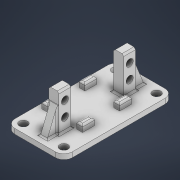
# Autodesk Inventor part: Servo mount
Saved by Autodesk Inventor 2021 (Build 250183000, 183)
## iProperties
Created: 2021-04-20
Part Number: Servo mount
Material: Generic
Document SubType Name: Modeling
Designer: allen
Density: 1 g/cm^3
Appearance: Default
Author: allen
Autodesk Inventor part; units mm, degrees
ref_plane "YZ Plane" through (0, 0, 0) normal (1, 0, 0) x (0, 1, 0)
ref_plane "XZ Plane" through (0, 0, 0) normal (0, 1, 0) x (-1, 0, 0)
ref_plane "XY Plane" through (0, 0, 0) normal (0, 0, 1) x (1, 0, 0)
sketch "Sketch1" plane through (0, 0, 0) normal (0, 1, 0) x (-1, 0, 0)
  line L0 (0, 0) -> (34, 0)
  line L1 (34, 0) -> (34, -65)
  line L2 (34, -65) -> (0, -65)
  line L3 (0, -65) -> (0, 0)
  dimension "d0" = 34
  dimension "d1" = 65
  constraints: 8 end point, 2 parallel, 1 horizontal, 1 perpendicular
  measures "d0" distance of L0.start L0.end
  measures "d1" distance of L2.end L0.start
extrude "Extrusion1" add sketch "Sketch1" along normal blind 3
sketch "Sketch2" plane through (0, 3, 0) normal (0, 1, 0) x (1, 0, 0)
  line L0 (-31, 11) -> (-3, 11) construction
  line L1 (-3, 11) -> (-3, 54) construction
  line L2 (-3, 54) -> (-31, 54) construction
  line L3 (-31, 54) -> (-31, 11) construction
  line L4 (0, 0) -> (0, 65) construction
  line L5 (-12.7, 11) -> (-10.4, 11) construction
  line L6 (-10.4, 11) -> (-10.4, 16.8) construction
  line L7 (-10.4, 16.8) -> (-12.7, 16.8) construction
  line L8 (-12.7, 16.8) -> (-12.7, 11) construction
  line L9 (0, 65) -> (-34, 65) construction
  line L10 (-12.7, 16.8) -> (-18.7, 16.8)
  line L11 (-18.7, 16.8) -> (-18.7, 9.8)
  line L12 (-18.7, 9.8) -> (-12.7, 9.8)
  line L13 (-12.7, 9.8) -> (-12.7, 16.8)
  line L14 (-6.9, 18) -> (-6.9, 25)
  line L15 (-6.9, 25) -> (-10.4, 25)
  line L16 (-27.5, 18) -> (-27.5, 25)
  line L17 (-27.5, 25) -> (-31, 25)
  line L18 (-31, 25) -> (-31, 18)
  line L19 (-31, 18) -> (-27.5, 18)
  line L20 (-10.4, 25) -> (-10.4, 18)
  line L21 (-10.4, 18) -> (-6.9, 18)
  line L22 (-3, 32.5) -> (-10.4, 32.5) construction
  point P0 (0, 32.5)
  point P1 (-17, 54)
  point P2 (-17, 65)
  point P3 (-12.7, 13.3)
  dimension "d5" = 5.8
  dimension "d6" = 7.4
  dimension "d7" = 2.3
  dimension "d8" = 28
  dimension "d11" = 6
  dimension "d23" = 7
  dimension "d24" = 7
  dimension "d25" = 3.5
  dimension "d26" = 7
  dimension "d27" = 3.5
  dimension "d30" = 7
  dimension "d67" = 19.2
  constraints: 42 end point, 7 parallel, 6 perpendicular, 5 horizontal, 5 midpoint, 3 collinear, 2 point on line, 1 horizontal alignment, 1 vertical, 1 vertical alignment
  measures "d5" distance between parallel lines of L7 L0
  measures "d6" distance between parallel lines of L1 L6
  measures "d7" distance of L6.end L7.end
  measures "d8" distance of L1.end L2.end
  measures "d11" distance of L7.end L10.end
  measures "d23" distance of L10.end L11.end
  measures "d24" distance of L14.start L14.end
  measures "d25" distance of L14.end L15.end
  measures "d26" distance of L16.start L16.end
  measures "d27" distance of L16.end L17.end
  measures "d30" distance between parallel lines of L0 L19
  measures "d67" distance from line of L22 point (-12.7, 13.3)
extrude "Extrusion2" add sketch "Sketch2" along normal blind 22 contours L13 L12 L11 L10
sketch "Sketch3" plane through (-12.7, 3, -9.8) normal (1, 0, 0) x (0, 0, -1)
  line L0 (0, 22) -> (7, 22) projected
  point P0 (-9.8, -3)
  point P1 (3.5, 16)
  point P2 (3.5, 7.4)
  point P3 (3.5, 22)
  dimension "d14" = 8.6
  dimension "d15" = 6
  constraints: 2 vertical alignment, 1 midpoint
  measures "d14" distance of point (3.5, 7.4) point (3.5, 16)
  measures "d15" distance of point (3.5, 22) point (3.5, 16)
hole "Hole1" at (-12.7, 19, -13.3) at (-12.7, 10.4, -13.3) direction (-1, 0, 0) diameter 4.2 end through all
extrude "Extrusion3" add sketch "Sketch2" along normal blind 3.75 contours L21 L20 L15 L14 | L19 L18 L17 L16
ref_plane "Work Plane1" through (-15.7, 3, -9.8) normal (1, 0, 0) x (0, 0, -1)
sketch "Sketch4" plane through (-15.7, 3, -9.8) normal (1, 0, 0) x (0, 0, -1)
  line L0 (0, 15) -> (-6, 0)
  line L1 (0, 0) -> (0, 22) construction
  line L2 (55.2, 0) -> (-9.8, 0) construction
  point P0 (-9.8, -3)
  dimension "d31" = 15
  dimension "d32" = 6
  constraints: 2 end point, 2 point on line
  measures "d31" distance from line of L2 L0.start
  measures "d32" distance of L1.start L0.end
extrude "Rib1" add sketch "Sketch4" along normal mid plane 4 rib yes fills toward (-2.9536, 7.4814) open curves L0
fillet "Fillet1" radius 1 19 edges at (-6.9, 6.75, -21.5) (-10.4, 6.75, -21.5) (-8.65, 6.75, -25) (-8.65, 6.75, -18) (-29.25, 6.75, -25) (-27.5, 6.75, -21.5) (-29.25, 6.75, -18) (-31, 6.75, -21.5) (-15.7, 3, -16.8) (-12.7, 3, -13.3) (-13.2, 3, -9.8) (-13.7, 3, -6.8) (-15.7, 3, -3.8) (-17.7, 3, -6.8) (-18.2, 3, -9.8) (-18.7, 3, -13.3) (-13.7, 10.5, -9.8) (-15.7, 18, -9.8) (-17.7, 10.5, -9.8)
chamfer "Chamfer1" distance 1 angle 45 2 edges at (-12.7, 25, -13.3) (-18.7, 25, -13.3)
ref_plane "Work Plane2" through (0, 0, -32.5) normal (0, 0, -1) x (-1, 0, 0)
mirror "Mirror2" about plane through (0, 0, -32.5) normal (0, 0, -1) of "Rib1", "Fillet1", "Chamfer1", "Extrusion3", "Hole1", "Extrusion2", "Extrusion1"
fillet "Fillet4" radius 5 4 edges at (-34, 1.5, 0) (-34, 1.5, -65) (0, 1.5, 0) (0, 1.5, -65)
sketch "Sketch7" plane through (0, 3, 0) normal (0, 1, 0) x (1, 0, 0)
  arc A0 (-34, 5) -> (-29, 0) centre (-29, 5) ccw projected
  arc A1 (-5, 0) -> (0, 5) centre (-5, 5) ccw projected
  arc A2 (0, 60) -> (-5, 65) centre (-5, 60) ccw projected
  arc A3 (-29, 65) -> (-34, 60) centre (-29, 60) ccw projected
  point P0 (0, 0)
  constraints: 4 coincident
hole "Hole4" at (-29, 3, -5) at (-5, 3, -5) at (-5, 3, -60) at (-29, 3, -60) direction (0, -1, 0) diameter 4.9 end through all
body "Solid1"
